Autodesk Inventor part; units mm, degrees
(part 9 of 13)
  line L3155 (8.6694, 25.137) -> (17.121, 25.137)
  arc A3155 (17.121, 25.137) -> (17.121, 25.263) centre (17.121, 25.2) ccw
  line L3156 (17.121, 25.263) -> (8.6694, 25.263)
  arc A3156 (8.6694, 25.263) -> (8.6694, 25.137) centre (8.6694, 25.2) ccw
  line L3157 (1.0789, 25.263) -> (6.8565, 25.263)
  arc A3157 (6.8565, 25.263) -> (6.8565, 25.389) centre (6.8565, 25.326) ccw
  line L3158 (6.8565, 25.389) -> (1.0789, 25.389)
  arc A3158 (1.0789, 25.389) -> (1.0789, 25.263) centre (1.0789, 25.326) ccw
  line L3159 (8.5434, 25.263) -> (17.121, 25.263)
  arc A3159 (17.121, 25.263) -> (17.121, 25.389) centre (17.121, 25.326) ccw
  line L3160 (17.121, 25.389) -> (8.5434, 25.389)
  arc A3160 (8.5434, 25.389) -> (8.5434, 25.263) centre (8.5434, 25.326) ccw
  line L3161 (1.0789, 25.389) -> (1.8946, 25.389)
  arc A3161 (1.8946, 25.389) -> (1.8946, 25.515) centre (1.8946, 25.452) ccw
  line L3162 (1.8946, 25.515) -> (1.0789, 25.515)
  arc A3162 (1.0789, 25.515) -> (1.0789, 25.389) centre (1.0789, 25.452) ccw
  line L3163 (2.9052, 25.389) -> (6.9825, 25.389)
  arc A3163 (6.9825, 25.389) -> (6.9825, 25.515) centre (6.9825, 25.452) ccw
  line L3164 (6.9825, 25.515) -> (2.9052, 25.515)
  arc A3164 (2.9052, 25.515) -> (2.9052, 25.389) centre (2.9052, 25.452) ccw
  line L3165 (8.4174, 25.389) -> (17.121, 25.389)
  arc A3165 (17.121, 25.389) -> (17.121, 25.515) centre (17.121, 25.452) ccw
  line L3166 (17.121, 25.515) -> (8.4174, 25.515)
  arc A3166 (8.4174, 25.515) -> (8.4174, 25.389) centre (8.4174, 25.452) ccw
  line L3167 (1.0789, 25.515) -> (1.6945, 25.515)
  arc A3167 (1.6945, 25.515) -> (1.6945, 25.641) centre (1.6945, 25.578) ccw
  line L3168 (1.6945, 25.641) -> (1.0789, 25.641)
  arc A3168 (1.0789, 25.641) -> (1.0789, 25.515) centre (1.0789, 25.578) ccw
  line L3169 (3.1054, 25.515) -> (7.2858, 25.515)
  arc A3169 (7.2858, 25.515) -> (7.2858, 25.641) centre (7.2858, 25.578) ccw
  line L3170 (7.2858, 25.641) -> (3.1054, 25.641)
  arc A3170 (3.1054, 25.641) -> (3.1054, 25.515) centre (3.1054, 25.578) ccw
  line L3171 (8.1142, 25.515) -> (17.121, 25.515)
  arc A3171 (17.121, 25.515) -> (17.121, 25.641) centre (17.121, 25.578) ccw
  line L3172 (17.121, 25.641) -> (8.1142, 25.641)
  arc A3172 (8.1142, 25.641) -> (8.1142, 25.515) centre (8.1142, 25.578) ccw
  line L3173 (1.0789, 25.641) -> (1.5685, 25.641)
  arc A3173 (1.5685, 25.641) -> (1.5685, 25.767) centre (1.5685, 25.704) ccw
  line L3174 (1.5685, 25.767) -> (1.0789, 25.767)
  arc A3174 (1.0789, 25.767) -> (1.0789, 25.641) centre (1.0789, 25.704) ccw
  line L3175 (3.2314, 25.641) -> (17.121, 25.641)
  arc A3175 (17.121, 25.641) -> (17.121, 25.767) centre (17.121, 25.704) ccw
  line L3176 (17.121, 25.767) -> (3.2314, 25.767)
  arc A3176 (3.2314, 25.767) -> (3.2314, 25.641) centre (3.2314, 25.704) ccw
  line L3177 (1.0789, 25.767) -> (1.4494, 25.767)
  arc A3177 (1.4494, 25.767) -> (1.4494, 25.893) centre (1.4494, 25.83) ccw
  line L3178 (1.4494, 25.893) -> (1.0789, 25.893)
  arc A3178 (1.0789, 25.893) -> (1.0789, 25.767) centre (1.0789, 25.83) ccw
  line L3179 (3.3504, 25.767) -> (17.121, 25.767)
  arc A3179 (17.121, 25.767) -> (17.121, 25.893) centre (17.121, 25.83) ccw
  line L3180 (17.121, 25.893) -> (3.3504, 25.893)
  arc A3180 (3.3504, 25.893) -> (3.3504, 25.767) centre (3.3504, 25.83) ccw
  line L3181 (1.0789, 25.893) -> (1.3972, 25.893)
  arc A3181 (1.3972, 25.893) -> (1.3972, 26.019) centre (1.3972, 25.956) ccw
  line L3182 (1.3972, 26.019) -> (1.0789, 26.019)
  arc A3182 (1.0789, 26.019) -> (1.0789, 25.893) centre (1.0789, 25.956) ccw
  line L3183 (3.4026, 25.893) -> (17.121, 25.893)
  arc A3183 (17.121, 25.893) -> (17.121, 26.019) centre (17.121, 25.956) ccw
  line L3184 (17.121, 26.019) -> (3.4026, 26.019)
  arc A3184 (3.4026, 26.019) -> (3.4026, 25.893) centre (3.4026, 25.956) ccw
  line L3185 (1.0789, 26.019) -> (1.3451, 26.019)
  arc A3185 (1.3451, 26.019) -> (1.3451, 26.145) centre (1.3451, 26.082) ccw
  line L3186 (1.3451, 26.145) -> (1.0789, 26.145)
  arc A3186 (1.0789, 26.145) -> (1.0789, 26.019) centre (1.0789, 26.082) ccw
  line L3187 (3.4547, 26.019) -> (17.121, 26.019)
  arc A3187 (17.121, 26.019) -> (17.121, 26.145) centre (17.121, 26.082) ccw
  line L3188 (17.121, 26.145) -> (3.4547, 26.145)
  arc A3188 (3.4547, 26.145) -> (3.4547, 26.019) centre (3.4547, 26.082) ccw
  line L3189 (1.0789, 26.145) -> (1.2929, 26.145)
  arc A3189 (1.2929, 26.145) -> (1.2929, 26.271) centre (1.2929, 26.208) ccw
  line L3190 (1.2929, 26.271) -> (1.0789, 26.271)
  arc A3190 (1.0789, 26.271) -> (1.0789, 26.145) centre (1.0789, 26.208) ccw
  line L3191 (3.5069, 26.145) -> (17.121, 26.145)
  arc A3191 (17.121, 26.145) -> (17.121, 26.271) centre (17.121, 26.208) ccw
  line L3192 (17.121, 26.271) -> (3.5069, 26.271)
  arc A3192 (3.5069, 26.271) -> (3.5069, 26.145) centre (3.5069, 26.208) ccw
  line L3193 (1.0789, 26.271) -> (1.2846, 26.271)
  arc A3193 (1.2846, 26.271) -> (1.2846, 26.397) centre (1.2846, 26.334) ccw
  line L3194 (1.2846, 26.397) -> (1.0789, 26.397)
  arc A3194 (1.0789, 26.397) -> (1.0789, 26.271) centre (1.0789, 26.334) ccw
  line L3195 (3.5153, 26.271) -> (17.121, 26.271)
  arc A3195 (17.121, 26.271) -> (17.121, 26.397) centre (17.121, 26.334) ccw
  line L3196 (17.121, 26.397) -> (3.5153, 26.397)
  arc A3196 (3.5153, 26.397) -> (3.5153, 26.271) centre (3.5153, 26.334) ccw
  line L3197 (1.0789, 26.397) -> (1.2846, 26.397)
  arc A3197 (1.2846, 26.397) -> (1.2846, 26.523) centre (1.2846, 26.46) ccw
  line L3198 (1.2846, 26.523) -> (1.0789, 26.523)
  arc A3198 (1.0789, 26.523) -> (1.0789, 26.397) centre (1.0789, 26.46) ccw
  line L3199 (3.5153, 26.397) -> (17.121, 26.397)
  arc A3199 (17.121, 26.397) -> (17.121, 26.523) centre (17.121, 26.46) ccw
  line L3200 (17.121, 26.523) -> (3.5153, 26.523)
  arc A3200 (3.5153, 26.523) -> (3.5153, 26.397) centre (3.5153, 26.46) ccw
  line L3201 (1.0789, 26.523) -> (1.2846, 26.523)
  arc A3201 (1.2846, 26.523) -> (1.2846, 26.649) centre (1.2846, 26.586) ccw
  line L3202 (1.2846, 26.649) -> (1.0789, 26.649)
  arc A3202 (1.0789, 26.649) -> (1.0789, 26.523) centre (1.0789, 26.586) ccw
  line L3203 (3.5153, 26.523) -> (17.121, 26.523)
  arc A3203 (17.121, 26.523) -> (17.121, 26.649) centre (17.121, 26.586) ccw
  line L3204 (17.121, 26.649) -> (3.5153, 26.649)
  arc A3204 (3.5153, 26.649) -> (3.5153, 26.523) centre (3.5153, 26.586) ccw
  line L3205 (1.0789, 26.649) -> (1.3013, 26.649)
  arc A3205 (1.3013, 26.649) -> (1.3013, 26.775) centre (1.3013, 26.712) ccw
  line L3206 (1.3013, 26.775) -> (1.0789, 26.775)
  arc A3206 (1.0789, 26.775) -> (1.0789, 26.649) centre (1.0789, 26.712) ccw
  line L3207 (3.4987, 26.649) -> (17.121, 26.649)
  arc A3207 (17.121, 26.649) -> (17.121, 26.775) centre (17.121, 26.712) ccw
  line L3208 (17.121, 26.775) -> (3.4987, 26.775)
  arc A3208 (3.4987, 26.775) -> (3.4987, 26.649) centre (3.4987, 26.712) ccw
  line L3209 (1.0789, 26.775) -> (1.3535, 26.775)
  arc A3209 (1.3535, 26.775) -> (1.3535, 26.901) centre (1.3535, 26.838) ccw
  line L3210 (1.3535, 26.901) -> (1.0789, 26.901)
  arc A3210 (1.0789, 26.901) -> (1.0789, 26.775) centre (1.0789, 26.838) ccw
  line L3211 (3.4465, 26.775) -> (17.121, 26.775)
  arc A3211 (17.121, 26.775) -> (17.121, 26.901) centre (17.121, 26.838) ccw
  line L3212 (17.121, 26.901) -> (3.4465, 26.901)
  arc A3212 (3.4465, 26.901) -> (3.4465, 26.775) centre (3.4465, 26.838) ccw
  line L3213 (1.0789, 26.901) -> (1.4057, 26.901)
  arc A3213 (1.4057, 26.901) -> (1.4057, 27.027) centre (1.4057, 26.964) ccw
  line L3214 (1.4057, 27.027) -> (1.0789, 27.027)
  arc A3214 (1.0789, 27.027) -> (1.0789, 26.901) centre (1.0789, 26.964) ccw
  line L3215 (3.3943, 26.901) -> (17.121, 26.901)
  arc A3215 (17.121, 26.901) -> (17.121, 27.027) centre (17.121, 26.964) ccw
  line L3216 (17.121, 27.027) -> (3.3943, 27.027)
  arc A3216 (3.3943, 27.027) -> (3.3943, 26.901) centre (3.3943, 26.964) ccw
  line L3217 (1.0789, 27.027) -> (1.4626, 27.027)
  arc A3217 (1.4626, 27.027) -> (1.4626, 27.153) centre (1.4626, 27.09) ccw
  line L3218 (1.4626, 27.153) -> (1.0789, 27.153)
  arc A3218 (1.0789, 27.153) -> (1.0789, 27.027) centre (1.0789, 27.09) ccw
  line L3219 (3.3373, 27.027) -> (17.121, 27.027)
  arc A3219 (17.121, 27.027) -> (17.121, 27.153) centre (17.121, 27.09) ccw
  line L3220 (17.121, 27.153) -> (3.3373, 27.153)
  arc A3220 (3.3373, 27.153) -> (3.3373, 27.027) centre (3.3373, 27.09) ccw
  line L3221 (1.0789, 27.153) -> (1.5886, 27.153)
  arc A3221 (1.5886, 27.153) -> (1.5886, 27.279) centre (1.5886, 27.216) ccw
  line L3222 (1.5886, 27.279) -> (1.0789, 27.279)
  arc A3222 (1.0789, 27.279) -> (1.0789, 27.153) centre (1.0789, 27.216) ccw
  line L3223 (3.2113, 27.153) -> (17.121, 27.153)
  arc A3223 (17.121, 27.153) -> (17.121, 27.279) centre (17.121, 27.216) ccw
  line L3224 (17.121, 27.279) -> (3.2113, 27.279)
  arc A3224 (3.2113, 27.279) -> (3.2113, 27.153) centre (3.2113, 27.216) ccw
  line L3225 (1.0789, 27.279) -> (1.7146, 27.279)
  arc A3225 (1.7146, 27.279) -> (1.7146, 27.405) centre (1.7146, 27.342) ccw
  line L3226 (1.7146, 27.405) -> (1.0789, 27.405)
  arc A3226 (1.0789, 27.405) -> (1.0789, 27.279) centre (1.0789, 27.342) ccw
  line L3227 (3.0853, 27.279) -> (17.121, 27.279)
  arc A3227 (17.121, 27.279) -> (17.121, 27.405) centre (17.121, 27.342) ccw
  line L3228 (17.121, 27.405) -> (3.0853, 27.405)
  arc A3228 (3.0853, 27.405) -> (3.0853, 27.279) centre (3.0853, 27.342) ccw
  line L3229 (1.0789, 27.405) -> (1.9432, 27.405)
  arc A3229 (1.9432, 27.405) -> (1.9432, 27.531) centre (1.9432, 27.468) ccw
  line L3230 (1.9432, 27.531) -> (1.0789, 27.531)
  arc A3230 (1.0789, 27.531) -> (1.0789, 27.405) centre (1.0789, 27.468) ccw
  line L3231 (2.8568, 27.405) -> (17.121, 27.405)
  arc A3231 (17.121, 27.405) -> (17.121, 27.531) centre (17.121, 27.468) ccw
  line L3232 (17.121, 27.531) -> (2.8568, 27.531)
  arc A3232 (2.8568, 27.531) -> (2.8568, 27.405) centre (2.8568, 27.468) ccw
  line L3233 (1.0789, 27.531) -> (17.121, 27.531)
  arc A3233 (17.121, 27.531) -> (17.121, 27.657) centre (17.121, 27.594) ccw
  line L3234 (17.121, 27.657) -> (1.0789, 27.657)
  arc A3234 (1.0789, 27.657) -> (1.0789, 27.531) centre (1.0789, 27.594) ccw
  line L3235 (1.0789, 27.657) -> (17.121, 27.657)
  arc A3235 (17.121, 27.657) -> (17.121, 27.783) centre (17.121, 27.72) ccw
  line L3236 (17.121, 27.783) -> (1.0789, 27.783)
  arc A3236 (1.0789, 27.783) -> (1.0789, 27.657) centre (1.0789, 27.72) ccw
  line L3237 (1.0789, 27.783) -> (17.121, 27.783)
  arc A3237 (17.121, 27.783) -> (17.121, 27.909) centre (17.121, 27.846) ccw
  line L3238 (17.121, 27.909) -> (1.0789, 27.909)
  arc A3238 (1.0789, 27.909) -> (1.0789, 27.783) centre (1.0789, 27.846) ccw
  line L3239 (1.0789, 27.909) -> (17.121, 27.909)
  arc A3239 (17.121, 27.909) -> (17.121, 28.035) centre (17.121, 27.972) ccw
  line L3240 (17.121, 28.035) -> (1.0789, 28.035)
  arc A3240 (1.0789, 28.035) -> (1.0789, 27.909) centre (1.0789, 27.972) ccw
  line L3241 (1.0789, 28.035) -> (7.4159, 28.035)
  arc A3241 (7.4159, 28.035) -> (7.4159, 28.161) centre (7.4159, 28.098) ccw
  line L3242 (7.4159, 28.161) -> (1.0789, 28.161)
  arc A3242 (1.0789, 28.161) -> (1.0789, 28.035) centre (1.0789, 28.098) ccw
  line L3243 (7.637, 28.035) -> (7.7628, 28.035)
  arc A3243 (7.7628, 28.035) -> (7.7628, 28.161) centre (7.7628, 28.098) ccw
  line L3244 (7.7628, 28.161) -> (7.637, 28.161)
  arc A3244 (7.637, 28.161) -> (7.637, 28.035) centre (7.637, 28.098) ccw
  line L3245 (7.9839, 28.035) -> (17.121, 28.035)
  arc A3245 (17.121, 28.035) -> (17.121, 28.161) centre (17.121, 28.098) ccw
  line L3246 (17.121, 28.161) -> (7.9839, 28.161)
  arc A3246 (7.9839, 28.161) -> (7.9839, 28.035) centre (7.9839, 28.098) ccw
  line L3247 (1.0789, 28.161) -> (7.1117, 28.161)
  arc A3247 (7.1117, 28.161) -> (7.1117, 28.287) centre (7.1117, 28.224) ccw
  line L3248 (7.1117, 28.287) -> (1.0789, 28.287)
  arc A3248 (1.0789, 28.287) -> (1.0789, 28.161) centre (1.0789, 28.224) ccw
  line L3249 (7.637, 28.161) -> (7.7628, 28.161)
  arc A3249 (7.7628, 28.161) -> (7.7628, 28.287) centre (7.7628, 28.224) ccw
  line L3250 (7.7628, 28.287) -> (7.637, 28.287)
  arc A3250 (7.637, 28.287) -> (7.637, 28.161) centre (7.637, 28.224) ccw
  line L3251 (8.2881, 28.161) -> (17.121, 28.161)
  arc A3251 (17.121, 28.161) -> (17.121, 28.287) centre (17.121, 28.224) ccw
  line L3252 (17.121, 28.287) -> (8.2881, 28.287)
  arc A3252 (8.2881, 28.287) -> (8.2881, 28.161) centre (8.2881, 28.224) ccw
  line L3253 (1.0789, 28.287) -> (6.8767, 28.287)
  arc A3253 (6.8767, 28.287) -> (6.8767, 28.413) centre (6.8767, 28.35) ccw
  line L3254 (6.8767, 28.413) -> (1.0789, 28.413)
  arc A3254 (1.0789, 28.413) -> (1.0789, 28.287) centre (1.0789, 28.35) ccw
  line L3255 (7.637, 28.287) -> (7.7628, 28.287)
  arc A3255 (7.7628, 28.287) -> (7.7628, 28.413) centre (7.7628, 28.35) ccw
  line L3256 (7.7628, 28.413) -> (7.637, 28.413)
  arc A3256 (7.637, 28.413) -> (7.637, 28.287) centre (7.637, 28.35) ccw
  line L3257 (8.5232, 28.287) -> (17.121, 28.287)
  arc A3257 (17.121, 28.287) -> (17.121, 28.413) centre (17.121, 28.35) ccw
  line L3258 (17.121, 28.413) -> (8.5232, 28.413)
  arc A3258 (8.5232, 28.413) -> (8.5232, 28.287) centre (8.5232, 28.35) ccw
  line L3259 (1.0789, 28.413) -> (6.7507, 28.413)
  arc A3259 (6.7507, 28.413) -> (6.7507, 28.539) centre (6.7507, 28.476) ccw
  line L3260 (6.7507, 28.539) -> (1.0789, 28.539)
  arc A3260 (1.0789, 28.539) -> (1.0789, 28.413) centre (1.0789, 28.476) ccw
  line L3261 (7.637, 28.413) -> (7.7628, 28.413)
  arc A3261 (7.7628, 28.413) -> (7.7628, 28.539) centre (7.7628, 28.476) ccw
  line L3262 (7.7628, 28.539) -> (7.637, 28.539)
  arc A3262 (7.637, 28.539) -> (7.637, 28.413) centre (7.637, 28.476) ccw
  line L3263 (8.6492, 28.413) -> (17.121, 28.413)
  arc A3263 (17.121, 28.413) -> (17.121, 28.539) centre (17.121, 28.476) ccw
  line L3264 (17.121, 28.539) -> (8.6492, 28.539)
  arc A3264 (8.6492, 28.539) -> (8.6492, 28.413) centre (8.6492, 28.476) ccw
  line L3265 (1.0789, 28.539) -> (6.6247, 28.539)
  arc A3265 (6.6247, 28.539) -> (6.6247, 28.665) centre (6.6247, 28.602) ccw
  line L3266 (6.6247, 28.665) -> (1.0789, 28.665)
  arc A3266 (1.0789, 28.665) -> (1.0789, 28.539) centre (1.0789, 28.602) ccw
  line L3267 (7.637, 28.539) -> (7.7628, 28.539)
  arc A3267 (7.7628, 28.539) -> (7.7628, 28.665) centre (7.7628, 28.602) ccw
  line L3268 (7.7628, 28.665) -> (7.637, 28.665)
  arc A3268 (7.637, 28.665) -> (7.637, 28.539) centre (7.637, 28.602) ccw
  line L3269 (8.7752, 28.539) -> (17.121, 28.539)
  arc A3269 (17.121, 28.539) -> (17.121, 28.665) centre (17.121, 28.602) ccw
  line L3270 (17.121, 28.665) -> (8.7752, 28.665)
  arc A3270 (8.7752, 28.665) -> (8.7752, 28.539) centre (8.7752, 28.602) ccw
  line L3271 (1.0789, 28.665) -> (6.5235, 28.665)
  arc A3271 (6.5235, 28.665) -> (6.5235, 28.791) centre (6.5235, 28.728) ccw
  line L3272 (6.5235, 28.791) -> (1.0789, 28.791)
  arc A3272 (1.0789, 28.791) -> (1.0789, 28.665) centre (1.0789, 28.728) ccw
  line L3273 (7.637, 28.665) -> (7.7628, 28.665)
  arc A3273 (7.7628, 28.665) -> (7.7628, 28.791) centre (7.7628, 28.728) ccw
  line L3274 (7.7628, 28.791) -> (7.637, 28.791)
  arc A3274 (7.637, 28.791) -> (7.637, 28.665) centre (7.637, 28.728) ccw
  line L3275 (8.8763, 28.665) -> (17.121, 28.665)
  arc A3275 (17.121, 28.665) -> (17.121, 28.791) centre (17.121, 28.728) ccw
  line L3276 (17.121, 28.791) -> (8.8763, 28.791)
  arc A3276 (8.8763, 28.791) -> (8.8763, 28.665) centre (8.8763, 28.728) ccw
  line L3277 (1.0789, 28.791) -> (1.8657, 28.791)
  arc A3277 (1.8657, 28.791) -> (1.8657, 28.917) centre (1.8657, 28.854) ccw
  line L3278 (1.8657, 28.917) -> (1.0789, 28.917)
  arc A3278 (1.0789, 28.917) -> (1.0789, 28.791) centre (1.0789, 28.854) ccw
  line L3279 (2.337, 28.791) -> (2.4628, 28.791)
  arc A3279 (2.4628, 28.791) -> (2.4628, 28.917) centre (2.4628, 28.854) ccw
  line L3280 (2.4628, 28.917) -> (2.337, 28.917)
  arc A3280 (2.337, 28.917) -> (2.337, 28.791) centre (2.337, 28.854) ccw
  line L3281 (2.9341, 28.791) -> (6.4713, 28.791)
  arc A3281 (6.4713, 28.791) -> (6.4713, 28.917) centre (6.4713, 28.854) ccw
  line L3282 (6.4713, 28.917) -> (2.9341, 28.917)
  arc A3282 (2.9341, 28.917) -> (2.9341, 28.791) centre (2.9341, 28.854) ccw
  line L3283 (7.637, 28.791) -> (7.7628, 28.791)
  arc A3283 (7.7628, 28.791) -> (7.7628, 28.917) centre (7.7628, 28.854) ccw
  line L3284 (7.7628, 28.917) -> (7.637, 28.917)
  arc A3284 (7.637, 28.917) -> (7.637, 28.791) centre (7.637, 28.854) ccw
  line L3285 (8.9285, 28.791) -> (17.121, 28.791)
  arc A3285 (17.121, 28.791) -> (17.121, 28.917) centre (17.121, 28.854) ccw
  line L3286 (17.121, 28.917) -> (8.9285, 28.917)
  arc A3286 (8.9285, 28.917) -> (8.9285, 28.791) centre (8.9285, 28.854) ccw
  line L3287 (1.0789, 28.917) -> (1.6489, 28.917)
  arc A3287 (1.6489, 28.917) -> (1.6489, 29.043) centre (1.6489, 28.98) ccw
  line L3288 (1.6489, 29.043) -> (1.0789, 29.043)
  arc A3288 (1.0789, 29.043) -> (1.0789, 28.917) centre (1.0789, 28.98) ccw
  line L3289 (2.337, 28.917) -> (2.4628, 28.917)
  arc A3289 (2.4628, 28.917) -> (2.4628, 29.043) centre (2.4628, 28.98) ccw
  line L3290 (2.4628, 29.043) -> (2.337, 29.043)
  arc A3290 (2.337, 29.043) -> (2.337, 28.917) centre (2.337, 28.98) ccw
  line L3291 (3.151, 28.917) -> (6.4191, 28.917)
  arc A3291 (6.4191, 28.917) -> (6.4191, 29.043) centre (6.4191, 28.98) ccw
  line L3292 (6.4191, 29.043) -> (3.151, 29.043)
  arc A3292 (3.151, 29.043) -> (3.151, 28.917) centre (3.151, 28.98) ccw
  line L3293 (7.637, 28.917) -> (7.7628, 28.917)
  arc A3293 (7.7628, 28.917) -> (7.7628, 29.043) centre (7.7628, 28.98) ccw
  line L3294 (7.7628, 29.043) -> (7.637, 29.043)
  arc A3294 (7.637, 29.043) -> (7.637, 28.917) centre (7.637, 28.98) ccw
  line L3295 (8.9807, 28.917) -> (17.121, 28.917)
  arc A3295 (17.121, 28.917) -> (17.121, 29.043) centre (17.121, 28.98) ccw
  line L3296 (17.121, 29.043) -> (8.9807, 29.043)
  arc A3296 (8.9807, 29.043) -> (8.9807, 28.917) centre (8.9807, 28.98) ccw
  line L3297 (1.0789, 29.043) -> (1.5229, 29.043)
  arc A3297 (1.5229, 29.043) -> (1.5229, 29.169) centre (1.5229, 29.106) ccw
  line L3298 (1.5229, 29.169) -> (1.0789, 29.169)
  arc A3298 (1.0789, 29.169) -> (1.0789, 29.043) centre (1.0789, 29.106) ccw
  line L3299 (2.337, 29.043) -> (2.4628, 29.043)
  arc A3299 (2.4628, 29.043) -> (2.4628, 29.169) centre (2.4628, 29.106) ccw
  line L3300 (2.4628, 29.169) -> (2.337, 29.169)
  arc A3300 (2.337, 29.169) -> (2.337, 29.043) centre (2.337, 29.106) ccw
  line L3301 (3.277, 29.043) -> (6.3669, 29.043)
  arc A3301 (6.3669, 29.043) -> (6.3669, 29.169) centre (6.3669, 29.106) ccw
  line L3302 (6.3669, 29.169) -> (3.277, 29.169)
  arc A3302 (3.277, 29.169) -> (3.277, 29.043) centre (3.277, 29.106) ccw
  line L3303 (7.637, 29.043) -> (7.7628, 29.043)
  arc A3303 (7.7628, 29.043) -> (7.7628, 29.169) centre (7.7628, 29.106) ccw
  line L3304 (7.7628, 29.169) -> (7.637, 29.169)
  arc A3304 (7.637, 29.169) -> (7.637, 29.043) centre (7.637, 29.106) ccw
  line L3305 (9.0329, 29.043) -> (17.121, 29.043)
  arc A3305 (17.121, 29.043) -> (17.121, 29.169) centre (17.121, 29.106) ccw
  line L3306 (17.121, 29.169) -> (9.0329, 29.169)
  arc A3306 (9.0329, 29.169) -> (9.0329, 29.043) centre (9.0329, 29.106) ccw
  line L3307 (1.0789, 29.169) -> (1.3969, 29.169)
  arc A3307 (1.3969, 29.169) -> (1.3969, 29.295) centre (1.3969, 29.232) ccw
  line L3308 (1.3969, 29.295) -> (1.0789, 29.295)
  arc A3308 (1.0789, 29.295) -> (1.0789, 29.169) centre (1.0789, 29.232) ccw
  line L3309 (2.337, 29.169) -> (2.4628, 29.169)
  arc A3309 (2.4628, 29.169) -> (2.4628, 29.295) centre (2.4628, 29.232) ccw
  line L3310 (2.4628, 29.295) -> (2.337, 29.295)
  arc A3310 (2.337, 29.295) -> (2.337, 29.169) centre (2.337, 29.232) ccw
  line L3311 (3.403, 29.169) -> (6.333, 29.169)
  arc A3311 (6.333, 29.169) -> (6.333, 29.295) centre (6.333, 29.232) ccw
  line L3312 (6.333, 29.295) -> (3.403, 29.295)
  arc A3312 (3.403, 29.295) -> (3.403, 29.169) centre (3.403, 29.232) ccw
  line L3313 (7.637, 29.169) -> (7.7628, 29.169)
  arc A3313 (7.7628, 29.169) -> (7.7628, 29.295) centre (7.7628, 29.232) ccw
  line L3314 (7.7628, 29.295) -> (7.637, 29.295)
  arc A3314 (7.637, 29.295) -> (7.637, 29.169) centre (7.637, 29.232) ccw
  line L3315 (9.0669, 29.169) -> (17.121, 29.169)
  arc A3315 (17.121, 29.169) -> (17.121, 29.295) centre (17.121, 29.232) ccw
  line L3316 (17.121, 29.295) -> (9.0669, 29.295)
  arc A3316 (9.0669, 29.295) -> (9.0669, 29.169) centre (9.0669, 29.232) ccw
  line L3317 (1.0789, 29.295) -> (1.3279, 29.295)
  arc A3317 (1.3279, 29.295) -> (1.3279, 29.421) centre (1.3279, 29.358) ccw
  line L3318 (1.3279, 29.421) -> (1.0789, 29.421)
  arc A3318 (1.0789, 29.421) -> (1.0789, 29.295) centre (1.0789, 29.358) ccw
  line L3319 (2.337, 29.295) -> (2.4628, 29.295)
  arc A3319 (2.4628, 29.295) -> (2.4628, 29.421) centre (2.4628, 29.358) ccw
  line L3320 (2.4628, 29.421) -> (2.337, 29.421)
  arc A3320 (2.337, 29.421) -> (2.337, 29.295) centre (2.337, 29.358) ccw
  line L3321 (3.4719, 29.295) -> (6.333, 29.295)
  arc A3321 (6.333, 29.295) -> (6.333, 29.421) centre (6.333, 29.358) ccw
  line L3322 (6.333, 29.421) -> (3.4719, 29.421)
  arc A3322 (3.4719, 29.421) -> (3.4719, 29.295) centre (3.4719, 29.358) ccw
  line L3323 (7.637, 29.295) -> (7.7628, 29.295)
  arc A3323 (7.7628, 29.295) -> (7.7628, 29.421) centre (7.7628, 29.358) ccw
  line L3324 (7.7628, 29.421) -> (7.637, 29.421)
  arc A3324 (7.637, 29.421) -> (7.637, 29.295) centre (7.637, 29.358) ccw
  line L3325 (9.0669, 29.295) -> (17.121, 29.295)
  arc A3325 (17.121, 29.295) -> (17.121, 29.421) centre (17.121, 29.358) ccw
  line L3326 (17.121, 29.421) -> (9.0669, 29.421)
  arc A3326 (9.0669, 29.421) -> (9.0669, 29.295) centre (9.0669, 29.358) ccw
  line L3327 (1.0789, 29.421) -> (1.2757, 29.421)
  arc A3327 (1.2757, 29.421) -> (1.2757, 29.547) centre (1.2757, 29.484) ccw
  line L3328 (1.2757, 29.547) -> (1.0789, 29.547)
  arc A3328 (1.0789, 29.547) -> (1.0789, 29.421) centre (1.0789, 29.484) ccw
  line L3329 (2.337, 29.421) -> (2.4628, 29.421)
  arc A3329 (2.4628, 29.421) -> (2.4628, 29.547) centre (2.4628, 29.484) ccw
  line L3330 (2.4628, 29.547) -> (2.337, 29.547)
  arc A3330 (2.337, 29.547) -> (2.337, 29.421) centre (2.337, 29.484) ccw
  line L3331 (3.5241, 29.421) -> (7.6365, 29.421)
  arc A3331 (7.6365, 29.421) -> (7.6365, 29.547) centre (7.6365, 29.484) ccw
  line L3332 (7.6365, 29.547) -> (3.5241, 29.547)
  arc A3332 (3.5241, 29.547) -> (3.5241, 29.421) centre (3.5241, 29.484) ccw
  line L3333 (7.7634, 29.421) -> (17.121, 29.421)
  arc A3333 (17.121, 29.421) -> (17.121, 29.547) centre (17.121, 29.484) ccw
  line L3334 (17.121, 29.547) -> (7.7634, 29.547)
  arc A3334 (7.7634, 29.547) -> (7.7634, 29.421) centre (7.7634, 29.484) ccw
  line L3335 (1.0789, 29.547) -> (1.2235, 29.547)
  arc A3335 (1.2235, 29.547) -> (1.2235, 29.673) centre (1.2235, 29.61) ccw
  line L3336 (1.2235, 29.673) -> (1.0789, 29.673)
  arc A3336 (1.0789, 29.673) -> (1.0789, 29.547) centre (1.0789, 29.61) ccw
  line L3337 (2.337, 29.547) -> (2.4628, 29.547)
  arc A3337 (2.4628, 29.547) -> (2.4628, 29.673) centre (2.4628, 29.61) ccw
  line L3338 (2.4628, 29.673) -> (2.337, 29.673)
  arc A3338 (2.337, 29.673) -> (2.337, 29.547) centre (2.337, 29.61) ccw
  line L3339 (3.5763, 29.547) -> (6.333, 29.547)
  arc A3339 (6.333, 29.547) -> (6.333, 29.673) centre (6.333, 29.61) ccw
  line L3340 (6.333, 29.673) -> (3.5763, 29.673)
  arc A3340 (3.5763, 29.673) -> (3.5763, 29.547) centre (3.5763, 29.61) ccw
  line L3341 (7.637, 29.547) -> (7.7628, 29.547)
  arc A3341 (7.7628, 29.547) -> (7.7628, 29.673) centre (7.7628, 29.61) ccw
  line L3342 (7.7628, 29.673) -> (7.637, 29.673)
  arc A3342 (7.637, 29.673) -> (7.637, 29.547) centre (7.637, 29.61) ccw
  line L3343 (9.0669, 29.547) -> (17.121, 29.547)
  arc A3343 (17.121, 29.547) -> (17.121, 29.673) centre (17.121, 29.61) ccw
  line L3344 (17.121, 29.673) -> (9.0669, 29.673)
  arc A3344 (9.0669, 29.673) -> (9.0669, 29.547) centre (9.0669, 29.61) ccw
  line L3345 (1.0789, 29.673) -> (1.183, 29.673)
  arc A3345 (1.183, 29.673) -> (1.183, 29.799) centre (1.183, 29.736) ccw
  line L3346 (1.183, 29.799) -> (1.0789, 29.799)
  arc A3346 (1.0789, 29.799) -> (1.0789, 29.673) centre (1.0789, 29.736) ccw
  line L3347 (2.337, 29.673) -> (2.4628, 29.673)
  arc A3347 (2.4628, 29.673) -> (2.4628, 29.799) centre (2.4628, 29.736) ccw
  line L3348 (2.4628, 29.799) -> (2.337, 29.799)
  arc A3348 (2.337, 29.799) -> (2.337, 29.673) centre (2.337, 29.736) ccw
  line L3349 (3.6169, 29.673) -> (6.3347, 29.673)
  arc A3349 (6.3347, 29.673) -> (6.3347, 29.799) centre (6.3347, 29.736) ccw
  line L3350 (6.3347, 29.799) -> (3.6169, 29.799)
  arc A3350 (3.6169, 29.799) -> (3.6169, 29.673) centre (3.6169, 29.736) ccw
  line L3351 (7.637, 29.673) -> (7.7628, 29.673)
  arc A3351 (7.7628, 29.673) -> (7.7628, 29.799) centre (7.7628, 29.736) ccw
  line L3352 (7.7628, 29.799) -> (7.637, 29.799)
  arc A3352 (7.637, 29.799) -> (7.637, 29.673) centre (7.637, 29.736) ccw
  line L3353 (9.0653, 29.673) -> (17.121, 29.673)
  arc A3353 (17.121, 29.673) -> (17.121, 29.799) centre (17.121, 29.736) ccw
  line L3354 (17.121, 29.799) -> (9.0653, 29.799)
  arc A3354 (9.0653, 29.799) -> (9.0653, 29.673) centre (9.0653, 29.736) ccw
  line L3355 (1.0789, 29.799) -> (1.183, 29.799)
  arc A3355 (1.183, 29.799) -> (1.183, 29.925) centre (1.183, 29.862) ccw
  line L3356 (1.183, 29.925) -> (1.0789, 29.925)
  arc A3356 (1.0789, 29.925) -> (1.0789, 29.799) centre (1.0789, 29.862) ccw
  line L3357 (2.337, 29.799) -> (2.4628, 29.799)
  arc A3357 (2.4628, 29.799) -> (2.4628, 29.925) centre (2.4628, 29.862) ccw
  line L3358 (2.4628, 29.925) -> (2.337, 29.925)
  arc A3358 (2.337, 29.925) -> (2.337, 29.799) centre (2.337, 29.862) ccw
  line L3359 (3.6169, 29.799) -> (6.3869, 29.799)
  arc A3359 (6.3869, 29.799) -> (6.3869, 29.925) centre (6.3869, 29.862) ccw
  line L3360 (6.3869, 29.925) -> (3.6169, 29.925)
  arc A3360 (3.6169, 29.925) -> (3.6169, 29.799) centre (3.6169, 29.862) ccw
  line L3361 (7.637, 29.799) -> (7.7628, 29.799)
  arc A3361 (7.7628, 29.799) -> (7.7628, 29.925) centre (7.7628, 29.862) ccw
  line L3362 (7.7628, 29.925) -> (7.637, 29.925)
  arc A3362 (7.637, 29.925) -> (7.637, 29.799) centre (7.637, 29.862) ccw
  line L3363 (9.0131, 29.799) -> (17.121, 29.799)
  arc A3363 (17.121, 29.799) -> (17.121, 29.925) centre (17.121, 29.862) ccw
  line L3364 (17.121, 29.925) -> (9.0131, 29.925)
  arc A3364 (9.0131, 29.925) -> (9.0131, 29.799) centre (9.0131, 29.862) ccw
  line L3365 (1.0789, 29.925) -> (2.3365, 29.925)
  arc A3365 (2.3365, 29.925) -> (2.3365, 30.051) centre (2.3365, 29.988) ccw
  line L3366 (2.3365, 30.051) -> (1.0789, 30.051)
  arc A3366 (1.0789, 30.051) -> (1.0789, 29.925) centre (1.0789, 29.988) ccw
  line L3367 (2.4634, 29.925) -> (6.4391, 29.925)
  arc A3367 (6.4391, 29.925) -> (6.4391, 30.051) centre (6.4391, 29.988) ccw
  line L3368 (6.4391, 30.051) -> (2.4634, 30.051)
  arc A3368 (2.4634, 30.051) -> (2.4634, 29.925) centre (2.4634, 29.988) ccw
  line L3369 (7.637, 29.925) -> (7.7628, 29.925)
  arc A3369 (7.7628, 29.925) -> (7.7628, 30.051) centre (7.7628, 29.988) ccw
  line L3370 (7.7628, 30.051) -> (7.637, 30.051)
  arc A3370 (7.637, 30.051) -> (7.637, 29.925) centre (7.637, 29.988) ccw
  line L3371 (8.9609, 29.925) -> (17.121, 29.925)
  arc A3371 (17.121, 29.925) -> (17.121, 30.051) centre (17.121, 29.988) ccw
  line L3372 (17.121, 30.051) -> (8.9609, 30.051)
  arc A3372 (8.9609, 30.051) -> (8.9609, 29.925) centre (8.9609, 29.988) ccw
  line L3373 (1.0789, 30.051) -> (1.183, 30.051)
  arc A3373 (1.183, 30.051) -> (1.183, 30.177) centre (1.183, 30.114) ccw
  line L3374 (1.183, 30.177) -> (1.0789, 30.177)
  arc A3374 (1.0789, 30.177) -> (1.0789, 30.051) centre (1.0789, 30.114) ccw
  line L3375 (2.337, 30.051) -> (2.4628, 30.051)
  arc A3375 (2.4628, 30.051) -> (2.4628, 30.177) centre (2.4628, 30.114) ccw
  line L3376 (2.4628, 30.177) -> (2.337, 30.177)
  arc A3376 (2.337, 30.177) -> (2.337, 30.051) centre (2.337, 30.114) ccw
  line L3377 (3.6169, 30.051) -> (6.4913, 30.051)
  arc A3377 (6.4913, 30.051) -> (6.4913, 30.177) centre (6.4913, 30.114) ccw
  line L3378 (6.4913, 30.177) -> (3.6169, 30.177)
  arc A3378 (3.6169, 30.177) -> (3.6169, 30.051) centre (3.6169, 30.114) ccw
  line L3379 (7.637, 30.051) -> (7.7628, 30.051)
  arc A3379 (7.7628, 30.051) -> (7.7628, 30.177) centre (7.7628, 30.114) ccw
  line L3380 (7.7628, 30.177) -> (7.637, 30.177)
  arc A3380 (7.637, 30.177) -> (7.637, 30.051) centre (7.637, 30.114) ccw
  line L3381 (8.9087, 30.051) -> (17.121, 30.051)
  arc A3381 (17.121, 30.051) -> (17.121, 30.177) centre (17.121, 30.114) ccw
  line L3382 (17.121, 30.177) -> (8.9087, 30.177)
  arc A3382 (8.9087, 30.177) -> (8.9087, 30.051) centre (8.9087, 30.114) ccw
  line L3383 (1.0789, 30.177) -> (1.2029, 30.177)
  arc A3383 (1.2029, 30.177) -> (1.2029, 30.303) centre (1.2029, 30.24) ccw
  line L3384 (1.2029, 30.303) -> (1.0789, 30.303)
  arc A3384 (1.0789, 30.303) -> (1.0789, 30.177) centre (1.0789, 30.24) ccw
  line L3385 (2.337, 30.177) -> (2.4628, 30.177)
  arc A3385 (2.4628, 30.177) -> (2.4628, 30.303) centre (2.4628, 30.24) ccw
  line L3386 (2.4628, 30.303) -> (2.337, 30.303)
  arc A3386 (2.337, 30.303) -> (2.337, 30.177) centre (2.337, 30.24) ccw
  line L3387 (3.5971, 30.177) -> (6.5468, 30.177)
  arc A3387 (6.5468, 30.177) -> (6.5468, 30.303) centre (6.5468, 30.24) ccw
  line L3388 (6.5468, 30.303) -> (3.5971, 30.303)
  arc A3388 (3.5971, 30.303) -> (3.5971, 30.177) centre (3.5971, 30.24) ccw
  line L3389 (7.637, 30.177) -> (7.7628, 30.177)
  arc A3389 (7.7628, 30.177) -> (7.7628, 30.303) centre (7.7628, 30.24) ccw
  line L3390 (7.7628, 30.303) -> (7.637, 30.303)
  arc A3390 (7.637, 30.303) -> (7.637, 30.177) centre (7.637, 30.24) ccw
  line L3391 (8.8531, 30.177) -> (17.121, 30.177)
  arc A3391 (17.121, 30.177) -> (17.121, 30.303) centre (17.121, 30.24) ccw
  line L3392 (17.121, 30.303) -> (8.8531, 30.303)
  arc A3392 (8.8531, 30.303) -> (8.8531, 30.177) centre (8.8531, 30.24) ccw
  line L3393 (1.0789, 30.303) -> (1.2551, 30.303)
  arc A3393 (1.2551, 30.303) -> (1.2551, 30.429) centre (1.2551, 30.366) ccw
  line L3394 (1.2551, 30.429) -> (1.0789, 30.429)
  arc A3394 (1.0789, 30.429) -> (1.0789, 30.303) centre (1.0789, 30.366) ccw
  line L3395 (2.337, 30.303) -> (2.4628, 30.303)
  arc A3395 (2.4628, 30.303) -> (2.4628, 30.429) centre (2.4628, 30.366) ccw
  line L3396 (2.4628, 30.429) -> (2.337, 30.429)
  arc A3396 (2.337, 30.429) -> (2.337, 30.303) centre (2.337, 30.366) ccw
  line L3397 (3.5449, 30.303) -> (6.6728, 30.303)
  arc A3397 (6.6728, 30.303) -> (6.6728, 30.429) centre (6.6728, 30.366) ccw
  line L3398 (6.6728, 30.429) -> (3.5449, 30.429)
  arc A3398 (3.5449, 30.429) -> (3.5449, 30.303) centre (3.5449, 30.366) ccw
  line L3399 (7.637, 30.303) -> (7.7628, 30.303)
  arc A3399 (7.7628, 30.303) -> (7.7628, 30.429) centre (7.7628, 30.366) ccw
  line L3400 (7.7628, 30.429) -> (7.637, 30.429)
  arc A3400 (7.637, 30.429) -> (7.637, 30.303) centre (7.637, 30.366) ccw
  line L3401 (8.7271, 30.303) -> (17.121, 30.303)
  arc A3401 (17.121, 30.303) -> (17.121, 30.429) centre (17.121, 30.366) ccw
  line L3402 (17.121, 30.429) -> (8.7271, 30.429)
  arc A3402 (8.7271, 30.429) -> (8.7271, 30.303) centre (8.7271, 30.366) ccw
  line L3403 (1.0789, 30.429) -> (1.3073, 30.429)
  arc A3403 (1.3073, 30.429) -> (1.3073, 30.555) centre (1.3073, 30.492) ccw
  line L3404 (1.3073, 30.555) -> (1.0789, 30.555)
  arc A3404 (1.0789, 30.555) -> (1.0789, 30.429) centre (1.0789, 30.492) ccw
  line L3405 (2.337, 30.429) -> (2.4628, 30.429)
  arc A3405 (2.4628, 30.429) -> (2.4628, 30.555) centre (2.4628, 30.492) ccw
  line L3406 (2.4628, 30.555) -> (2.337, 30.555)
  arc A3406 (2.337, 30.555) -> (2.337, 30.429) centre (2.337, 30.492) ccw
  line L3407 (3.4927, 30.429) -> (6.7988, 30.429)
  arc A3407 (6.7988, 30.429) -> (6.7988, 30.555) centre (6.7988, 30.492) ccw
  line L3408 (6.7988, 30.555) -> (3.4927, 30.555)
  arc A3408 (3.4927, 30.555) -> (3.4927, 30.429) centre (3.4927, 30.492) ccw
  line L3409 (7.637, 30.429) -> (7.7628, 30.429)
  arc A3409 (7.7628, 30.429) -> (7.7628, 30.555) centre (7.7628, 30.492) ccw
  line L3410 (7.7628, 30.555) -> (7.637, 30.555)
  arc A3410 (7.637, 30.555) -> (7.637, 30.429) centre (7.637, 30.492) ccw
  line L3411 (8.6011, 30.429) -> (17.121, 30.429)
  arc A3411 (17.121, 30.429) -> (17.121, 30.555) centre (17.121, 30.492) ccw
  line L3412 (17.121, 30.555) -> (8.6011, 30.555)
  arc A3412 (8.6011, 30.555) -> (8.6011, 30.429) centre (8.6011, 30.492) ccw
  line L3413 (1.0789, 30.555) -> (1.3595, 30.555)
  arc A3413 (1.3595, 30.555) -> (1.3595, 30.681) centre (1.3595, 30.618) ccw
  line L3414 (1.3595, 30.681) -> (1.0789, 30.681)
  arc A3414 (1.0789, 30.681) -> (1.0789, 30.555) centre (1.0789, 30.618) ccw
  line L3415 (2.337, 30.555) -> (2.4628, 30.555)
  arc A3415 (2.4628, 30.555) -> (2.4628, 30.681) centre (2.4628, 30.618) ccw
  line L3416 (2.4628, 30.681) -> (2.337, 30.681)
  arc A3416 (2.337, 30.681) -> (2.337, 30.555) centre (2.337, 30.618) ccw
  line L3417 (3.4405, 30.555) -> (6.9248, 30.555)
  arc A3417 (6.9248, 30.555) -> (6.9248, 30.681) centre (6.9248, 30.618) ccw
  line L3418 (6.9248, 30.681) -> (3.4405, 30.681)
  arc A3418 (3.4405, 30.681) -> (3.4405, 30.555) centre (3.4405, 30.618) ccw
  line L3419 (7.637, 30.555) -> (7.7628, 30.555)
  arc A3419 (7.7628, 30.555) -> (7.7628, 30.681) centre (7.7628, 30.618) ccw
  line L3420 (7.7628, 30.681) -> (7.637, 30.681)
  arc A3420 (7.637, 30.681) -> (7.637, 30.555) centre (7.637, 30.618) ccw
  line L3421 (8.4751, 30.555) -> (17.121, 30.555)
  arc A3421 (17.121, 30.555) -> (17.121, 30.681) centre (17.121, 30.618) ccw
  line L3422 (17.121, 30.681) -> (8.4751, 30.681)
  arc A3422 (8.4751, 30.681) -> (8.4751, 30.555) centre (8.4751, 30.618) ccw
  line L3423 (1.0789, 30.681) -> (1.473, 30.681)
  arc A3423 (1.473, 30.681) -> (1.473, 30.807) centre (1.473, 30.744) ccw
  line L3424 (1.473, 30.807) -> (1.0789, 30.807)
  arc A3424 (1.0789, 30.807) -> (1.0789, 30.681) centre (1.0789, 30.744) ccw
  line L3425 (2.337, 30.681) -> (2.4628, 30.681)
  arc A3425 (2.4628, 30.681) -> (2.4628, 30.807) centre (2.4628, 30.744) ccw
  line L3426 (2.4628, 30.807) -> (2.337, 30.807)
  arc A3426 (2.337, 30.807) -> (2.337, 30.681) centre (2.337, 30.744) ccw
  line L3427 (3.3269, 30.681) -> (7.2279, 30.681)
  arc A3427 (7.2279, 30.681) -> (7.2279, 30.807) centre (7.2279, 30.744) ccw
  line L3428 (7.2279, 30.807) -> (3.3269, 30.807)
  arc A3428 (3.3269, 30.807) -> (3.3269, 30.681) centre (3.3269, 30.744) ccw
  line L3429 (7.637, 30.681) -> (7.7628, 30.681)
  arc A3429 (7.7628, 30.681) -> (7.7628, 30.807) centre (7.7628, 30.744) ccw
  line L3430 (7.7628, 30.807) -> (7.637, 30.807)
  arc A3430 (7.637, 30.807) -> (7.637, 30.681) centre (7.637, 30.744) ccw
  line L3431 (8.1721, 30.681) -> (17.121, 30.681)
  arc A3431 (17.121, 30.681) -> (17.121, 30.807) centre (17.121, 30.744) ccw
  line L3432 (17.121, 30.807) -> (8.1721, 30.807)
  arc A3432 (8.1721, 30.807) -> (8.1721, 30.681) centre (8.1721, 30.744) ccw
  line L3433 (1.0789, 30.807) -> (1.599, 30.807)
  arc A3433 (1.599, 30.807) -> (1.599, 30.933) centre (1.599, 30.87) ccw
  line L3434 (1.599, 30.933) -> (1.0789, 30.933)
  arc A3434 (1.0789, 30.933) -> (1.0789, 30.807) centre (1.0789, 30.87) ccw
  line L3435 (2.337, 30.807) -> (2.4628, 30.807)
  arc A3435 (2.4628, 30.807) -> (2.4628, 30.933) centre (2.4628, 30.87) ccw
  line L3436 (2.4628, 30.933) -> (2.337, 30.933)
  arc A3436 (2.337, 30.933) -> (2.337, 30.807) centre (2.337, 30.87) ccw
  line L3437 (3.2009, 30.807) -> (17.121, 30.807)
  arc A3437 (17.121, 30.807) -> (17.121, 30.933) centre (17.121, 30.87) ccw
  line L3438 (17.121, 30.933) -> (3.2009, 30.933)
  arc A3438 (3.2009, 30.933) -> (3.2009, 30.807) centre (3.2009, 30.87) ccw
  line L3439 (1.0789, 30.933) -> (1.7454, 30.933)
  arc A3439 (1.7454, 30.933) -> (1.7454, 31.059) centre (1.7454, 30.996) ccw
  line L3440 (1.7454, 31.059) -> (1.0789, 31.059)
  arc A3440 (1.0789, 31.059) -> (1.0789, 30.933) centre (1.0789, 30.996) ccw
  line L3441 (2.337, 30.933) -> (2.4628, 30.933)
  arc A3441 (2.4628, 30.933) -> (2.4628, 31.059) centre (2.4628, 30.996) ccw
  line L3442 (2.4628, 31.059) -> (2.337, 31.059)
  arc A3442 (2.337, 31.059) -> (2.337, 30.933) centre (2.337, 30.996) ccw
  line L3443 (3.0546, 30.933) -> (17.121, 30.933)
  arc A3443 (17.121, 30.933) -> (17.121, 31.059) centre (17.121, 30.996) ccw
  line L3444 (17.121, 31.059) -> (3.0546, 31.059)
  arc A3444 (3.0546, 31.059) -> (3.0546, 30.933) centre (3.0546, 30.996) ccw
  line L3445 (1.0789, 31.059) -> (2.0495, 31.059)
  arc A3445 (2.0495, 31.059) -> (2.0495, 31.185) centre (2.0495, 31.122) ccw
  line L3446 (2.0495, 31.185) -> (1.0789, 31.185)
  arc A3446 (1.0789, 31.185) -> (1.0789, 31.059) centre (1.0789, 31.122) ccw
  line L3447 (2.337, 31.059) -> (2.4628, 31.059)
  arc A3447 (2.4628, 31.059) -> (2.4628, 31.185) centre (2.4628, 31.122) ccw
  line L3448 (2.4628, 31.185) -> (2.337, 31.185)
  arc A3448 (2.337, 31.185) -> (2.337, 31.059) centre (2.337, 31.122) ccw
  line L3449 (2.7505, 31.059) -> (17.121, 31.059)
  arc A3449 (17.121, 31.059) -> (17.121, 31.185) centre (17.121, 31.122) ccw
  line L3450 (17.121, 31.185) -> (2.7505, 31.185)
  arc A3450 (2.7505, 31.185) -> (2.7505, 31.059) centre (2.7505, 31.122) ccw
  line L3451 (1.0789, 31.185) -> (17.121, 31.185)
  arc A3451 (17.121, 31.185) -> (17.121, 31.311) centre (17.121, 31.248) ccw
  line L3452 (17.121, 31.311) -> (1.0789, 31.311)
  arc A3452 (1.0789, 31.311) -> (1.0789, 31.185) centre (1.0789, 31.248) ccw
  line L3453 (1.0789, 31.311) -> (17.121, 31.311)
  arc A3453 (17.121, 31.311) -> (17.121, 31.437) centre (17.121, 31.374) ccw
  line L3454 (17.121, 31.437) -> (1.0789, 31.437)
  arc A3454 (1.0789, 31.437) -> (1.0789, 31.311) centre (1.0789, 31.374) ccw
  line L3455 (1.0789, 31.437) -> (17.121, 31.437)
  arc A3455 (17.121, 31.437) -> (17.121, 31.563) centre (17.121, 31.5) ccw
  line L3456 (17.121, 31.563) -> (1.0789, 31.563)
  arc A3456 (1.0789, 31.563) -> (1.0789, 31.437) centre (1.0789, 31.5) ccw
  line L3457 (1.0789, 31.563) -> (17.121, 31.563)
  arc A3457 (17.121, 31.563) -> (17.121, 31.689) centre (17.121, 31.626) ccw
  line L3458 (17.121, 31.689) -> (1.0789, 31.689)
  arc A3458 (1.0789, 31.689) -> (1.0789, 31.563) centre (1.0789, 31.626) ccw
  line L3459 (1.0789, 31.689) -> (17.121, 31.689)
  arc A3459 (17.121, 31.689) -> (17.121, 31.815) centre (17.121, 31.752) ccw
  line L3460 (17.121, 31.815) -> (1.0789, 31.815)
  arc A3460 (1.0789, 31.815) -> (1.0789, 31.689) centre (1.0789, 31.752) ccw
  line L3461 (1.0789, 31.815) -> (17.121, 31.815)
  arc A3461 (17.121, 31.815) -> (17.121, 31.941) centre (17.121, 31.878) ccw
  line L3462 (17.121, 31.941) -> (1.0789, 31.941)
  arc A3462 (1.0789, 31.941) -> (1.0789, 31.815) centre (1.0789, 31.878) ccw
  line L3463 (1.0789, 31.941) -> (17.121, 31.941)
  arc A3463 (17.121, 31.941) -> (17.121, 32.067) centre (17.121, 32.004) ccw
  line L3464 (17.121, 32.067) -> (1.0789, 32.067)
  arc A3464 (1.0789, 32.067) -> (1.0789, 31.941) centre (1.0789, 32.004) ccw
  line L3465 (1.0789, 32.067) -> (17.121, 32.067)
  arc A3465 (17.121, 32.067) -> (17.121, 32.193) centre (17.121, 32.13) ccw
  line L3466 (17.121, 32.193) -> (1.0789, 32.193)
  arc A3466 (1.0789, 32.193) -> (1.0789, 32.067) centre (1.0789, 32.13) ccw
  line L3467 (1.0789, 32.193) -> (17.121, 32.193)
  arc A3467 (17.121, 32.193) -> (17.121, 32.319) centre (17.121, 32.256) ccw
  line L3468 (17.121, 32.319) -> (1.0789, 32.319)
  arc A3468 (1.0789, 32.319) -> (1.0789, 32.193) centre (1.0789, 32.256) ccw
  line L3469 (1.0789, 32.319) -> (2.0636, 32.319)
  arc A3469 (2.0636, 32.319) -> (2.0636, 32.445) centre (2.0636, 32.382) ccw
  line L3470 (2.0636, 32.445) -> (1.0789, 32.445)
  arc A3470 (1.0789, 32.445) -> (1.0789, 32.319) centre (1.0789, 32.382) ccw
  line L3471 (2.7362, 32.319) -> (17.121, 32.319)
  arc A3471 (17.121, 32.319) -> (17.121, 32.445) centre (17.121, 32.382) ccw
  line L3472 (17.121, 32.445) -> (2.7362, 32.445)
  arc A3472 (2.7362, 32.445) -> (2.7362, 32.319) centre (2.7362, 32.382) ccw
  line L3473 (1.0789, 32.445) -> (1.7645, 32.445)
  arc A3473 (1.7645, 32.445) -> (1.7645, 32.571) centre (1.7645, 32.508) ccw
  line L3474 (1.7645, 32.571) -> (1.0789, 32.571)
  arc A3474 (1.0789, 32.571) -> (1.0789, 32.445) centre (1.0789, 32.508) ccw
  line L3475 (3.0354, 32.445) -> (17.121, 32.445)
  arc A3475 (17.121, 32.445) -> (17.121, 32.571) centre (17.121, 32.508) ccw
  line L3476 (17.121, 32.571) -> (3.0354, 32.571)
  arc A3476 (3.0354, 32.571) -> (3.0354, 32.445) centre (3.0354, 32.508) ccw
  line L3477 (1.0789, 32.571) -> (1.6385, 32.571)
  arc A3477 (1.6385, 32.571) -> (1.6385, 32.697) centre (1.6385, 32.634) ccw
  line L3478 (1.6385, 32.697) -> (1.0789, 32.697)
  arc A3478 (1.0789, 32.697) -> (1.0789, 32.571) centre (1.0789, 32.634) ccw
  line L3479 (3.1614, 32.571) -> (17.121, 32.571)
  arc A3479 (17.121, 32.571) -> (17.121, 32.697) centre (17.121, 32.634) ccw
  line L3480 (17.121, 32.697) -> (3.1614, 32.697)
  arc A3480 (3.1614, 32.697) -> (3.1614, 32.571) centre (3.1614, 32.634) ccw
  line L3481 (1.0789, 32.697) -> (1.5125, 32.697)
  arc A3481 (1.5125, 32.697) -> (1.5125, 32.823) centre (1.5125, 32.76) ccw
  line L3482 (1.5125, 32.823) -> (1.0789, 32.823)
  arc A3482 (1.0789, 32.823) -> (1.0789, 32.697) centre (1.0789, 32.76) ccw
  line L3483 (3.2874, 32.697) -> (17.121, 32.697)
  arc A3483 (17.121, 32.697) -> (17.121, 32.823) centre (17.121, 32.76) ccw
  line L3484 (17.121, 32.823) -> (3.2874, 32.823)
  arc A3484 (3.2874, 32.823) -> (3.2874, 32.697) centre (3.2874, 32.76) ccw
  line L3485 (1.0789, 32.823) -> (1.4262, 32.823)
  arc A3485 (1.4262, 32.823) -> (1.4262, 32.949) centre (1.4262, 32.886) ccw
  line L3486 (1.4262, 32.949) -> (1.0789, 32.949)
  arc A3486 (1.0789, 32.949) -> (1.0789, 32.823) centre (1.0789, 32.886) ccw
  line L3487 (3.3736, 32.823) -> (17.121, 32.823)
  arc A3487 (17.121, 32.823) -> (17.121, 32.949) centre (17.121, 32.886) ccw
  line L3488 (17.121, 32.949) -> (3.3736, 32.949)
  arc A3488 (3.3736, 32.949) -> (3.3736, 32.823) centre (3.3736, 32.886) ccw
  line L3489 (1.0789, 32.949) -> (1.374, 32.949)
  arc A3489 (1.374, 32.949) -> (1.374, 33.075) centre (1.374, 33.012) ccw
  line L3490 (1.374, 33.075) -> (1.0789, 33.075)
  arc A3490 (1.0789, 33.075) -> (1.0789, 32.949) centre (1.0789, 33.012) ccw
  line L3491 (3.4258, 32.949) -> (17.121, 32.949)
  arc A3491 (17.121, 32.949) -> (17.121, 33.075) centre (17.121, 33.012) ccw
  line L3492 (17.121, 33.075) -> (3.4258, 33.075)
  arc A3492 (3.4258, 33.075) -> (3.4258, 32.949) centre (3.4258, 33.012) ccw
  line L3493 (1.0789, 33.075) -> (1.3219, 33.075)
  arc A3493 (1.3219, 33.075) -> (1.3219, 33.201) centre (1.3219, 33.138) ccw
  line L3494 (1.3219, 33.201) -> (1.0789, 33.201)
  arc A3494 (1.0789, 33.201) -> (1.0789, 33.075) centre (1.0789, 33.138) ccw
  line L3495 (3.4779, 33.075) -> (17.121, 33.075)
  arc A3495 (17.121, 33.075) -> (17.121, 33.201) centre (17.121, 33.138) ccw
  line L3496 (17.121, 33.201) -> (3.4779, 33.201)
  arc A3496 (3.4779, 33.201) -> (3.4779, 33.075) centre (3.4779, 33.138) ccw
  line L3497 (1.0789, 33.201) -> (1.2846, 33.201)
  arc A3497 (1.2846, 33.201) -> (1.2846, 33.327) centre (1.2846, 33.264) ccw
  line L3498 (1.2846, 33.327) -> (1.0789, 33.327)
  arc A3498 (1.0789, 33.327) -> (1.0789, 33.201) centre (1.0789, 33.264) ccw
  line L3499 (3.5153, 33.201) -> (17.121, 33.201)
  arc A3499 (17.121, 33.201) -> (17.121, 33.327) centre (17.121, 33.264) ccw
  line L3500 (17.121, 33.327) -> (3.5153, 33.327)
  arc A3500 (3.5153, 33.327) -> (3.5153, 33.201) centre (3.5153, 33.264) ccw
  line L3501 (1.0789, 33.327) -> (1.2846, 33.327)
  arc A3501 (1.2846, 33.327) -> (1.2846, 33.453) centre (1.2846, 33.39) ccw
  line L3502 (1.2846, 33.453) -> (1.0789, 33.453)
  arc A3502 (1.0789, 33.453) -> (1.0789, 33.327) centre (1.0789, 33.39) ccw
  line L3503 (3.5153, 33.327) -> (7.1695, 33.327)
  arc A3503 (7.1695, 33.327) -> (7.1695, 33.453) centre (7.1695, 33.39) ccw
  line L3504 (7.1695, 33.453) -> (3.5153, 33.453)
  arc A3504 (3.5153, 33.453) -> (3.5153, 33.327) centre (3.5153, 33.39) ccw
  line L3505 (8.2303, 33.327) -> (17.121, 33.327)
  arc A3505 (17.121, 33.327) -> (17.121, 33.453) centre (17.121, 33.39) ccw
  line L3506 (17.121, 33.453) -> (8.2303, 33.453)
  arc A3506 (8.2303, 33.453) -> (8.2303, 33.327) centre (8.2303, 33.39) ccw
  line L3507 (1.0789, 33.453) -> (1.2846, 33.453)
  arc A3507 (1.2846, 33.453) -> (1.2846, 33.579) centre (1.2846, 33.516) ccw
  line L3508 (1.2846, 33.579) -> (1.0789, 33.579)
  arc A3508 (1.0789, 33.579) -> (1.0789, 33.453) centre (1.0789, 33.516) ccw
  line L3509 (3.5153, 33.453) -> (6.9344, 33.453)
  arc A3509 (6.9344, 33.453) -> (6.9344, 33.579) centre (6.9344, 33.516) ccw
  line L3510 (6.9344, 33.579) -> (3.5153, 33.579)
  arc A3510 (3.5153, 33.579) -> (3.5153, 33.453) centre (3.5153, 33.516) ccw
  line L3511 (8.4655, 33.453) -> (17.121, 33.453)
  arc A3511 (17.121, 33.453) -> (17.121, 33.579) centre (17.121, 33.516) ccw
  line L3512 (17.121, 33.579) -> (8.4655, 33.579)
  arc A3512 (8.4655, 33.579) -> (8.4655, 33.453) centre (8.4655, 33.516) ccw
  line L3513 (1.0789, 33.579) -> (1.2846, 33.579)
  arc A3513 (1.2846, 33.579) -> (1.2846, 33.705) centre (1.2846, 33.642) ccw
  line L3514 (1.2846, 33.705) -> (1.0789, 33.705)
  arc A3514 (1.0789, 33.705) -> (1.0789, 33.579) centre (1.0789, 33.642) ccw
  line L3515 (3.5153, 33.579) -> (6.8084, 33.579)
  arc A3515 (6.8084, 33.579) -> (6.8084, 33.705) centre (6.8084, 33.642) ccw
  line L3516 (6.8084, 33.705) -> (3.5153, 33.705)
  arc A3516 (3.5153, 33.705) -> (3.5153, 33.579) centre (3.5153, 33.642) ccw
  line L3517 (8.5915, 33.579) -> (17.121, 33.579)
  arc A3517 (17.121, 33.579) -> (17.121, 33.705) centre (17.121, 33.642) ccw
  line L3518 (17.121, 33.705) -> (8.5915, 33.705)
  arc A3518 (8.5915, 33.705) -> (8.5915, 33.579) centre (8.5915, 33.642) ccw
  line L3519 (1.0789, 33.705) -> (1.3245, 33.705)
  arc A3519 (1.3245, 33.705) -> (1.3245, 33.831) centre (1.3245, 33.768) ccw
  line L3520 (1.3245, 33.831) -> (1.0789, 33.831)
  arc A3520 (1.0789, 33.831) -> (1.0789, 33.705) centre (1.0789, 33.768) ccw
  line L3521 (3.4755, 33.705) -> (6.6824, 33.705)
  arc A3521 (6.6824, 33.705) -> (6.6824, 33.831) centre (6.6824, 33.768) ccw
  line L3522 (6.6824, 33.831) -> (3.4755, 33.831)
  arc A3522 (3.4755, 33.831) -> (3.4755, 33.705) centre (3.4755, 33.768) ccw
  line L3523 (8.7175, 33.705) -> (17.121, 33.705)
  arc A3523 (17.121, 33.705) -> (17.121, 33.831) centre (17.121, 33.768) ccw
  line L3524 (17.121, 33.831) -> (8.7175, 33.831)
  arc A3524 (8.7175, 33.831) -> (8.7175, 33.705) centre (8.7175, 33.768) ccw
  line L3525 (1.0789, 33.831) -> (1.3767, 33.831)
  arc A3525 (1.3767, 33.831) -> (1.3767, 33.957) centre (1.3767, 33.894) ccw
  line L3526 (1.3767, 33.957) -> (1.0789, 33.957)
  arc A3526 (1.0789, 33.957) -> (1.0789, 33.831) centre (1.0789, 33.894) ccw
  line L3527 (3.4233, 33.831) -> (6.5978, 33.831)
  arc A3527 (6.5978, 33.831) -> (6.5978, 33.957) centre (6.5978, 33.894) ccw
  line L3528 (6.5978, 33.957) -> (3.4233, 33.957)
  arc A3528 (3.4233, 33.957) -> (3.4233, 33.831) centre (3.4233, 33.894) ccw
  line L3529 (8.802, 33.831) -> (17.121, 33.831)
  arc A3529 (17.121, 33.831) -> (17.121, 33.957) centre (17.121, 33.894) ccw
  line L3530 (17.121, 33.957) -> (8.802, 33.957)
  arc A3530 (8.802, 33.957) -> (8.802, 33.831) centre (8.802, 33.894) ccw
  line L3531 (1.0789, 33.957) -> (1.4289, 33.957)
  arc A3531 (1.4289, 33.957) -> (1.4289, 34.083) centre (1.4289, 34.02) ccw
  line L3532 (1.4289, 34.083) -> (1.0789, 34.083)
  arc A3532 (1.0789, 34.083) -> (1.0789, 33.957) centre (1.0789, 34.02) ccw
  line L3533 (3.3711, 33.957) -> (6.5456, 33.957)
  arc A3533 (6.5456, 33.957) -> (6.5456, 34.083) centre (6.5456, 34.02) ccw
  line L3534 (6.5456, 34.083) -> (3.3711, 34.083)
  arc A3534 (3.3711, 34.083) -> (3.3711, 33.957) centre (3.3711, 34.02) ccw
  line L3535 (8.8542, 33.957) -> (17.121, 33.957)
  arc A3535 (17.121, 33.957) -> (17.121, 34.083) centre (17.121, 34.02) ccw
  line L3536 (17.121, 34.083) -> (8.8542, 34.083)
  arc A3536 (8.8542, 34.083) -> (8.8542, 33.957) centre (8.8542, 34.02) ccw
  line L3537 (1.0789, 34.083) -> (1.5186, 34.083)
  arc A3537 (1.5186, 34.083) -> (1.5186, 34.209) centre (1.5186, 34.146) ccw
  line L3538 (1.5186, 34.209) -> (1.0789, 34.209)
  arc A3538 (1.0789, 34.209) -> (1.0789, 34.083) centre (1.0789, 34.146) ccw
  line L3539 (3.2813, 34.083) -> (6.4934, 34.083)
  arc A3539 (6.4934, 34.083) -> (6.4934, 34.209) centre (6.4934, 34.146) ccw
  line L3540 (6.4934, 34.209) -> (3.2813, 34.209)
  arc A3540 (3.2813, 34.209) -> (3.2813, 34.083) centre (3.2813, 34.146) ccw
  line L3541 (8.9064, 34.083) -> (17.121, 34.083)
  arc A3541 (17.121, 34.083) -> (17.121, 34.209) centre (17.121, 34.146) ccw
  line L3542 (17.121, 34.209) -> (8.9064, 34.209)
  arc A3542 (8.9064, 34.209) -> (8.9064, 34.083) centre (8.9064, 34.146) ccw
  line L3543 (1.0789, 34.209) -> (1.6446, 34.209)
  arc A3543 (1.6446, 34.209) -> (1.6446, 34.335) centre (1.6446, 34.272) ccw
  line L3544 (1.6446, 34.335) -> (1.0789, 34.335)
  arc A3544 (1.0789, 34.335) -> (1.0789, 34.209) centre (1.0789, 34.272) ccw
  line L3545 (3.1553, 34.209) -> (6.4413, 34.209)
  arc A3545 (6.4413, 34.209) -> (6.4413, 34.335) centre (6.4413, 34.272) ccw
  line L3546 (6.4413, 34.335) -> (3.1553, 34.335)
  arc A3546 (3.1553, 34.335) -> (3.1553, 34.209) centre (3.1553, 34.272) ccw
  line L3547 (8.9585, 34.209) -> (17.121, 34.209)
  arc A3547 (17.121, 34.209) -> (17.121, 34.335) centre (17.121, 34.272) ccw
  line L3548 (17.121, 34.335) -> (8.9585, 34.335)
  arc A3548 (8.9585, 34.335) -> (8.9585, 34.209) centre (8.9585, 34.272) ccw
  line L3549 (1.0789, 34.335) -> (1.7742, 34.335)
  arc A3549 (1.7742, 34.335) -> (1.7742, 34.461) centre (1.7742, 34.398) ccw
  line L3550 (1.7742, 34.461) -> (1.0789, 34.461)